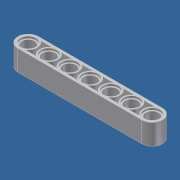
# Autodesk Inventor part: 7M Beam
Saved by Autodesk Inventor 2016 SP1 (Build 200210100, 210)
## iProperties
Created: 2014-02-10
Part Number: 7M Beam
Document SubType Name: Modeling
Designer: jleonard
Density: 1 g/cm^3
Material: Generic
Appearance: Default
Author: jleonard
Autodesk Inventor part; units mm, degrees
ref_plane "YZ Plane" through (0, 0, 0) normal (1, 0, 0) x (0, 1, 0)
ref_plane "XZ Plane" through (0, 0, 0) normal (0, 1, 0) x (-1, 0, 0)
ref_plane "XY Plane" through (0, 0, 0) normal (0, 0, 1) x (1, 0, 0)
sketch "Sketch2" plane through (0, 0, 0) normal (0, 0, 1) x (1, 0, 0)
  arc A0 (-24, 4) -> (-24, -4) centre (-24, 0) ccw
  arc A1 (24, -4) -> (24, 4) centre (24, 0) ccw
  line L0 (-24, 4) -> (24, 4)
  line L1 (-24, -4) -> (24, -4)
  line L2 (-39.2, 0) -> (39.2, 0) projected
  line L3 (0, -5.6) -> (0, 5.6) projected
  point P0 (0, 0)
  dimension "d0" = 4
  dimension "d1" = 4
  dimension "d2" = 48
  dimension "d3" = 0
  dimension "d4" = 24
  dimension "d9" = 180
  dimension "d10" = 0
  dimension "d98" = 48
  constraints: 6 point on circle, 4 end point, 2 centre point, 2 point on line, 2 tangent
  measures "d0" radius of A0
  measures "d1" radius of A1
  measures "d2" distance of A1.centre A0.centre
  measures "d3" distance from line of A0.centre L2
  measures "d4" distance from line of A0.centre L3
  measures "d9" angle of L0 L2
  measures "d10" distance from line of L2 A1.centre
  measures "d98" distance of L1.start L1.end
extrude "Extrusion1" add sketch "Sketch2" along normal blind 8
sketch "Sketch11" plane through (0, 0, 8) normal (0, 0, 1) x (1, 0, 0)
  arc A0 (-24, 4) -> (-24, -4) centre (-24, 0) ccw projected
  circle A1 centre (-24, 0) radius 2.5
  line L0 (-39.2, 0) -> (39.2, 0) projected
  circle A2 centre (-16, 0) radius 2.5
  circle A3 centre (-8, 0) radius 2.5
  circle A4 centre (0, 0) radius 2.5
  circle A5 centre (8, 0) radius 2.5
  circle A6 centre (16, 0) radius 2.5
  circle A7 centre (24, 0) radius 2.5
  dimension "d99" = 5
  dimension "d105" = 8
  constraints: 7 centre point, 1 coincident, 1 horizontal, 12 other
  measures "d99" diameter of A1
  measures "d105" distance of A1.centre A2.centre
extrude "Extrusion10" cut sketch "Sketch11" against normal through all
sketch "Sketch12" plane through (0, 0, 8) normal (0, 0, 1) x (1, 0, 0)
  circle A0 centre (24, 0) radius 2.5 projected
  circle A1 centre (16, 0) radius 2.5 projected
  circle A2 centre (8, 0) radius 2.5 projected
  circle A3 centre (0, 0) radius 2.5 projected
  circle A4 centre (-8, 0) radius 2.5 projected
  circle A5 centre (-16, 0) radius 2.5 projected
  circle A6 centre (-24, 0) radius 2.5 projected
  arc A7 (-24, 4) -> (-24, -4) centre (-24, 0) ccw projected
  circle A8 centre (-24, 0) radius 3
  line L0 (-39.2, 0) -> (39.2, 0) projected
  circle A9 centre (-16, 0) radius 3
  circle A10 centre (-8, 0) radius 3
  circle A11 centre (0, 0) radius 3
  circle A12 centre (8, 0) radius 3
  circle A13 centre (16, 0) radius 3
  circle A14 centre (24, 0) radius 3
  dimension "d109" = 6
  dimension "d115" = 8
  constraints: 7 centre point, 1 coincident, 1 horizontal, 12 other
  measures "d109" diameter of A8
  measures "d115" distance of A8.centre A9.centre
extrude "Extrusion11" cut sketch "Sketch12" against normal blind 0.8 contours L0 A14 A0 | A0 L0 A14 | A8 L0 A6 | L0 A6 A8 | A9 L0 A5 | L0 A5 A9 | A10 L0 A4 | L0 A4 A10 | A11 L0 A3 | L0 A3 A11 | A12 L0 A2 | L0 A2 A12 | A13 L0 A1 | L0 A1 A13
sketch "Sketch13" plane through (0, 0, 0) normal (0, 0, -1) x (-1, 0, 0)
  circle A0 centre (-24, 0) radius 2.5 projected
  circle A1 centre (-16, 0) radius 2.5 projected
  circle A2 centre (-8, 0) radius 2.5 projected
  circle A3 centre (0, 0) radius 2.5 projected
  circle A4 centre (8, 0) radius 2.5 projected
  circle A5 centre (16, 0) radius 2.5 projected
  circle A6 centre (24, 0) radius 2.5 projected
  arc A7 (-24, 4) -> (-24, -4) centre (-24, 0) ccw projected
  circle A8 centre (-24, 0) radius 3
  line L0 (39.2, 0) -> (-39.2, 0) projected
  circle A9 centre (-16, 0) radius 3
  circle A10 centre (-8, 0) radius 3
  circle A11 centre (0, 0) radius 3
  circle A12 centre (8, 0) radius 3
  circle A13 centre (16, 0) radius 3
  circle A14 centre (24, 0) radius 3
  dimension "d119" = 6
  dimension "d125" = 8
  constraints: 7 centre point, 1 coincident, 1 horizontal, 12 other
  measures "d119" diameter of A8
  measures "d125" distance of A8.centre A9.centre
extrude "Extrusion12" cut sketch "Sketch13" against normal blind 0.8 contours L0 A8 A0 | A0 L0 A8 | A14 L0 A6 | L0 A6 A14 | A13 L0 A5 | L0 A5 A13 | A12 L0 A4 | L0 A4 A12 | A11 L0 A3 | L0 A3 A11 | A10 L0 A2 | L0 A2 A10 | A9 L0 A1 | L0 A1 A9
sketch "Sketch14" plane through (0, 0, 8) normal (0, 0, 1) x (1, 0, 0)
  circle A0 centre (-24, 0) radius 3 projected
  circle A1 centre (-16, 0) radius 3 projected
  arc A2 (-24, 4) -> (-24, -4) centre (-24, 0) ccw projected
  line L0 (-24, 4) -> (24, 4) projected
  arc A3 (-22.1972, -3) -> (-22.1972, 3) centre (-24, 0) ccw
  line L1 (-22.1972, 3) -> (-17.8028, 3)
  line L2 (-22.1972, -3) -> (-17.8028, -3)
  arc A4 (-17.8028, 3) -> (-17.8028, -3) centre (-16, 0) ccw
  line L3 (-39.2, 0) -> (39.2, 0) projected
  arc A5 (-14.1972, -3) -> (-14.1972, 3) centre (-16, 0) ccw
  line L4 (-14.1972, 3) -> (-9.8028, 3)
  line L5 (-14.1972, -3) -> (-9.8028, -3)
  arc A6 (-9.8028, 3) -> (-9.8028, -3) centre (-8, 0) ccw
  arc A7 (-6.1972, -3) -> (-6.1972, 3) centre (-8, 0) ccw
  line L6 (-6.1972, 3) -> (-1.8028, 3)
  line L7 (-6.1972, -3) -> (-1.8028, -3)
  arc A8 (-1.8028, 3) -> (-1.8028, -3) centre (0, 0) ccw
  arc A9 (1.8028, -3) -> (1.8028, 3) centre (0, 0) ccw
  line L8 (1.8028, 3) -> (6.1972, 3)
  line L9 (1.8028, -3) -> (6.1972, -3)
  arc A10 (6.1972, 3) -> (6.1972, -3) centre (8, 0) ccw
  arc A11 (9.8028, -3) -> (9.8028, 3) centre (8, 0) ccw
  line L10 (9.8028, 3) -> (14.1972, 3)
  line L11 (9.8028, -3) -> (14.1972, -3)
  arc A12 (14.1972, 3) -> (14.1972, -3) centre (16, 0) ccw
  arc A13 (17.8028, -3) -> (17.8028, 3) centre (16, 0) ccw
  line L12 (17.8028, 3) -> (22.1972, 3)
  line L13 (17.8028, -3) -> (22.1972, -3)
  arc A14 (22.1972, 3) -> (22.1972, -3) centre (24, 0) ccw
  dimension "d129" = 7
  dimension "d131" = 7
  dimension "d137" = 8
  constraints: 24 end point, 24 point on circle, 12 centre point, 2 coincident, 2 parallel, 2 tangent, 1 horizontal, 50 other
  measures "d129" diameter of A3
  measures "d131" diameter of A4
  measures "d137" distance of L1.start L4.start
extrude "Extrusion13" cut sketch "Sketch14" against normal through all contours A13 L12 A14 L3 | L3 A14 L13 A13 | A11 L10 A12 L3 | L3 A12 L11 A11 | A9 L8 A10 L3 | L3 A10 L9 A9 | A7 L6 A8 L3 | L3 A8 L7 A7 | A5 L4 A6 L3 | L3 A6 L5 A5 | A3 L1 A4 L3 | L3 A4 L2 A3
body "Solid1"
